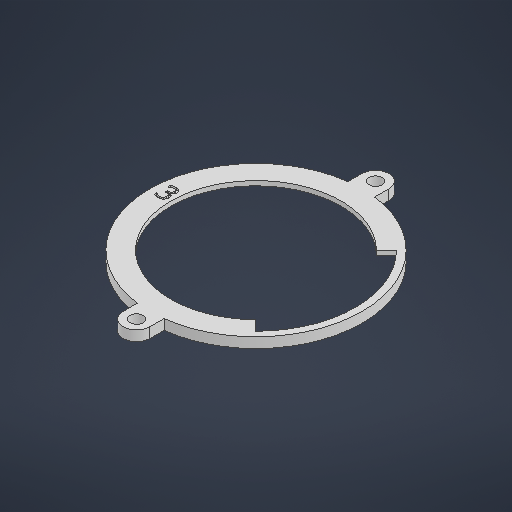
# Autodesk Inventor part: speaker clamp v1
Saved by Autodesk Inventor 2026.1 (Build 301233020, 233B)
## iProperties
Created: 2026-03-18
Part Number: speaker clamp v1
Material: Generic
Document SubType Name: Modeling
Designer: stoof
Density: 1 g/cm^3
Appearance: Default
Author: stoof
Autodesk Inventor part; units mm, degrees
ref_plane "YZ Plane" through (0, 0, 0) normal (1, 0, 0) x (0, 1, 0)
ref_plane "XZ Plane" through (0, 0, 0) normal (0, 1, 0) x (-1, 0, 0)
ref_plane "XY Plane" through (0, 0, 0) normal (0, 0, 1) x (1, 0, 0)
sketch "Sketch1" plane through (0, 0, 0) normal (0, 1, 0) x (-1, 0, 0)
  circle A0 centre (0, 0) radius 17 construction
  circle A1 centre (0, 0) radius 15
  circle A2 centre (0, 0) radius 18.7
  line L0 (0, 0) -> (-13.2229, 13.2229)
  line L1 (0, 0) -> (17, 0) construction
  line L2 (0, 0) -> (-13.2229, -13.2229)
  line L3 (0, 0) -> (17, 0) construction
  arc A3 (-12.3744, 12.3744) -> (-12.3744, -12.3744) centre (0, 0) ccw
  point P0 (-10.6066, -10.6066)
  point P1 (-10.6066, 10.6066)
  dimension "d0" = 34
  dimension "d1" = 2
  dimension "d2" = 1.7
  dimension "d14" = 135
  dimension "d15" = 135
  dimension "d17" = 35
  constraints: 8 end point, 4 point on circle, 3 centre point, 2 coincident, 2 horizontal, 2 point on line, 1 horizontal alignment, 2 other
  measures "d14" angle of L1 L0
  measures "d15" angle of L2 L3
  measures "d17" diameter of A3
extrude "Extrusion1" add sketch "Sketch1" along normal blind 0.8 contours A1 L0 A2 L2 | A1 L2 A3 L0 | A3 L2 A2 L0
sketch "Sketch2" plane through (0, 0, 0) normal (0, -1, 0) x (1, 0, 0)
  circle A0 centre (0, 0) radius 18.7 projected
  circle A1 centre (0, 0) radius 17.5
  dimension "d5" = 1.2
  constraints: 1 centre point
  measures "d5" radial gap between concentric circles of A0 A1
extrude "Extrusion2" add sketch "Sketch2" along normal blind 1
extrude "Extrusion5" cut sketch "Sketch1" along normal blind 1 contours A1 L2 A3 L0
sketch "Sketch3" plane through (0, 0.8, 0) normal (0, 1, 0) x (1, 0, 0)
  circle A0 centre (0, 0) radius 18.7 projected
  circle A1 centre (0, 21.05) radius 1.15
  circle A2 centre (0, 21.05) radius 2.35
  line L0 (2.35, 21.05) -> (2.35, 18.5518)
  line L1 (-2.35, 21.05) -> (-2.35, 18.5518)
  line L2 (0, 0) -> (1.9485, 0)
  circle A3 centre (0, 0) radius 18.7
  circle A4 centre (0, -21.05) radius 1.15
  circle A5 centre (0, -21.05) radius 2.35
  line L3 (2.35, -21.05) -> (2.35, -18.5518)
  line L4 (-2.35, -21.05) -> (-2.35, -18.5518)
  dimension "d8" = 2.3
  dimension "d9" = 1.2
  constraints: 10 end point, 8 point on circle, 5 centre point, 5 symmetric about line, 3 tangent, 2 vertical, 1 horizontal, 1 vertical alignment, 3 other
  measures "d8" diameter of A1
  measures "d9" radial gap between concentric circles of A1 A2
extrude "Extrusion3" add sketch "Sketch3" against normal up to surface (1.8 mm away) contours A0 A2 L0 | L3 A5 A0 | A0 L1 A2 | A2 | A5 L4 A0 | A5
sketch "Sketch4" plane through (0, 0.8, 0) normal (0, 1, 0) x (1, 0, 0)
  line L0 (-17.6802, 2.5436) -> (-15.393, 2.5436) construction
  line L1 (-15.393, 2.5436) -> (-15.393, -0.5686) construction
  line L2 (-15.393, -0.5686) -> (-17.6802, -0.5686) construction
  line L3 (-17.6802, -0.5686) -> (-17.6802, 2.5436) construction
  spline S0 degree 2 poles (-16.6354, 2.1904) (-16.7466, 2.1904) (-16.9664, 2.136) (-17.0726, 2.0941) knots 0 0 0 1 2 2 2
  spline S1 degree 2 poles (-17.0726, 2.0941) (-17.1714, 2.0521) (-17.3171, 1.9631) (-17.3739, 1.9236) knots 0 0 0 1 2 2 2
  line L4 (-17.3739, 1.9236) -> (-17.3986, 1.9236)
  line L5 (-17.3986, 1.9236) -> (-17.3986, 2.3559)
  spline S2 degree 2 poles (-17.3986, 2.3559) (-17.2653, 2.4275) (-16.8083, 2.5436) (-16.6033, 2.5436) knots 0 0 0 1 2 2 2
  spline S3 degree 2 poles (-16.6033, 2.5436) (-16.3958, 2.5436) (-16.0871, 2.4596) (-15.9611, 2.3707) knots 0 0 0 1 2 2 2
  spline S4 degree 2 poles (-15.9611, 2.3707) (-15.8277, 2.2744) (-15.6894, 1.9953) (-15.6894, 1.8075) knots 0 0 0 1 2 2 2
  spline S5 degree 2 poles (-15.6894, 1.8075) (-15.6894, 1.5556) (-16.0204, 1.1752) (-16.2525, 1.1258) knots 0 0 0 1 2 2 2
  line L6 (-16.2525, 1.1258) -> (-16.2525, 1.0962)
  spline S6 degree 2 poles (-16.2525, 1.0962) (-16.1562, 1.0764) (-15.9364, 0.9875) (-15.8425, 0.8986) knots 0 0 0 1 2 2 2
  spline S7 degree 2 poles (-15.8425, 0.8986) (-15.7487, 0.8121) (-15.6301, 0.5355) (-15.6301, 0.3354) knots 0 0 0 1 2 2 2
  spline S8 degree 2 poles (-15.6301, 0.3354) (-15.6301, 0.1304) (-15.7709, -0.2179) (-15.8993, -0.3513) knots 0 0 0 1 2 2 2
  spline S9 degree 2 poles (-15.8993, -0.3513) (-16.0327, -0.4896) (-16.4106, -0.6328) (-16.6502, -0.6328) knots 0 0 0 1 2 2 2
  spline S10 degree 2 poles (-16.6502, -0.6328) (-16.8799, -0.6328) (-17.3295, -0.5217) (-17.4826, -0.4451) knots 0 0 0 1 2 2 2
  line L7 (-17.4826, -0.4451) -> (-17.4826, -0.0129)
  line L8 (-17.4826, -0.0129) -> (-17.453, -0.0129)
  spline S11 degree 2 poles (-17.453, -0.0129) (-17.3245, -0.1067) (-16.8898, -0.2796) (-16.6749, -0.2796) knots 0 0 0 1 2 2 2
  spline S12 degree 2 poles (-16.6749, -0.2796) (-16.5489, -0.2796) (-16.297, -0.2006) (-16.213, -0.1092) knots 0 0 0 1 2 2 2
  spline S13 degree 2 poles (-16.213, -0.1092) (-16.1315, -0.0178) (-16.0451, 0.1996) (-16.0451, 0.365) knots 0 0 0 1 2 2 2
  spline S14 degree 2 poles (-16.0451, 0.365) (-16.0451, 0.5305) (-16.1414, 0.7454) (-16.2278, 0.8072) knots 0 0 0 1 2 2 2
  spline S15 degree 2 poles (-16.2278, 0.8072) (-16.3143, 0.8689) (-16.5489, 0.9159) (-16.6873, 0.9159) knots 0 0 0 1 2 2 2
  line L9 (-16.6873, 0.9159) -> (-16.8602, 0.9159)
  line L10 (-16.8602, 0.9159) -> (-16.8602, 1.2542)
  line L11 (-16.8602, 1.2542) -> (-16.7243, 1.2542)
  spline S16 degree 2 poles (-16.7243, 1.2542) (-16.4501, 1.2542) (-16.1043, 1.5161) (-16.1043, 1.7655) knots 0 0 0 1 2 2 2
  spline S17 degree 2 poles (-16.1043, 1.7655) (-16.1043, 1.8816) (-16.1933, 2.0471) (-16.2649, 2.0965) knots 0 0 0 1 2 2 2
  spline S18 degree 2 poles (-16.2649, 2.0965) (-16.3415, 2.1484) (-16.5292, 2.1904) (-16.6354, 2.1904) knots 0 0 0 1 2 2 2
  point P0 (0, 0)
  dimension "d1" = 2
  constraints: 2 other
extrude "Extrusion4" cut sketch "Sketch4" against normal blind 0.4
body "Solid1"
